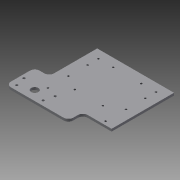
# Autodesk Inventor part: backplate
Saved by Autodesk Inventor 2013 (Build 170138000, 138)
## iProperties
Created: 2012-12-03
Part Number: backplate
Material: Generic
Document SubType Name: Sheet Metal
Designer: Istvan
Density: 1 g/cm^3
Sheet Metal Rule: Default
Flat Pattern Width: 24.13 cm
Flat Pattern Length: 20.32 cm
Flat Pattern Area: 490.322 cm^2
Sheet Metal Width: 9.500 in
Sheet Metal Length: 8.000 in
Sheet Metal Area: 76.000 in^2
Mass: 348.987 g
Surface Area: 1192.6 cm^2
Volume: 348.987 cm^3
Author: Istvan
Autodesk Inventor part; units mm, degrees
ref_plane "YZ Plane" through (0, 0, 0) normal (1, 0, 0) x (0, 1, 0)
ref_plane "XZ Plane" through (0, 0, 0) normal (0, 1, 0) x (-1, 0, 0)
ref_plane "XY Plane" through (0, 0, 0) normal (0, 0, 1) x (1, 0, 0)
sketch "Sketch1" plane through (0, 0, 0) normal (0, 1, 0) x (-1, 0, 0)
  line L0 (0, 0) -> (203.2, 0)
  line L1 (203.2, 0) -> (203.2, 114.3)
  line L2 (76.2, 165.1) -> (0, 165.1)
  line L3 (0, 165.1) -> (0, 0)
  line L4 (76.2, 165.1) -> (76.2, 190.5)
  line L5 (88.9, 203.2) -> (228.6, 203.2)
  arc A0 (63.5, 165.1) -> (76.2, 177.8) centre (63.5, 177.8) ccw
  arc A1 (241.3, 190.5) -> (228.6, 203.2) centre (228.6, 190.5) ccw
  arc A2 (88.9, 203.2) -> (76.2, 190.5) centre (88.9, 190.5) ccw
  line L6 (146.05, 0) -> (57.15, 0)
  line L7 (215.9, 127) -> (228.6, 127)
  line L8 (241.3, 139.7) -> (241.3, 190.5)
  arc A3 (215.9, 127) -> (203.2, 114.3) centre (215.9, 114.3) ccw
  arc A4 (228.6, 127) -> (241.3, 139.7) centre (228.6, 139.7) ccw
  point P0 (76.2, 203.2)
  point P1 (241.3, 127)
  dimension "d64" = 38.1
  dimension "d67" = 12.7
  dimension "d69" = 12.7
  dimension "d105" = 76.2
  dimension "d106" = 12.7
  dimension "d108" = 203.2
  dimension "d109" = 127
  dimension "d110" = 165.1
  dimension "d111" = 38.1
  constraints: 18 end point, 10 point on circle, 10 tangent, 6 point on line, 5 centre point, 3 horizontal, 2 equal radius, 2 parallel, 2 perpendicular, 1 midpoint
  measures "d64" distance of L2.start point (76.2, 203.2)
  measures "d67" radius of A0
  measures "d69" radius of A1
  measures "d105" distance between parallel lines of L3 L4
  measures "d106" radius of A3
  measures "d108" distance between parallel lines of L1 L3
  measures "d109" distance between parallel lines of L0 L7
  measures "d110" distance from line of L0.start L2
  measures "d111" distance between parallel lines of L8 L1
extrude "Plate2" add sketch "Sketch1" along normal blind 6.35
sketch "Sketch5" plane through (0, 6.35, 0) normal (0, 1, 0) x (1, 0, 0)
  line L0 (-203.2, -114.3) -> (-203.2, 0) projected
  line L1 (0, 0) -> (0, -165.1) projected
  line L2 (-203.2, 0) -> (0, 0) projected
  point P0 (-203.2, -165.1)
  point P1 (-177.8, -22.225)
  point P2 (-25.4, -22.225)
  point P3 (-25.4, -155.575)
  point P4 (-177.8, -155.575)
  point P5 (-177.8, -50.8)
  point P6 (-177.8, -101.6)
  point P7 (-25.4, -50.8)
  point P8 (-25.4, -101.6)
  point P9 (-203.2, -203.2)
  point P10 (-138.684, -22.225)
  point P11 (-64.516, -22.225)
  point P12 (-138.684, -123.825)
  point P13 (-64.516, -123.825)
  dimension "d27" = 25.4
  dimension "d28" = 25.4
  dimension "d30" = 133.35
  dimension "d62" = 22.225
  dimension "d89" = 50.8
  dimension "d90" = 50.8
  dimension "d91" = 25.4
  dimension "d93" = 152.4
  dimension "d94" = 25.4
  dimension "d147" = 64.516
  dimension "d148" = 64.516
  dimension "d149" = 101.6
  constraints: 7 horizontal alignment, 6 vertical alignment
  measures "d27" distance from line of L0 point (-177.8, -22.225)
  measures "d28" distance from line of L1 point (-25.4, -22.225)
  measures "d30" distance of point (-177.8, -155.575) point (-177.8, -22.225)
  measures "d62" distance from line of L2 point (-177.8, -22.225)
  measures "d89" distance from line of L2 point (-177.8, -50.8)
  measures "d90" distance of point (-177.8, -50.8) point (-177.8, -101.6)
  measures "d91" distance from line of L0 point (-177.8, -101.6)
  measures "d93" distance of point (-25.4, -50.8) point (-177.8, -50.8)
  measures "d94" distance from line of L1 point (-25.4, -50.8)
  measures "d147" distance from line of point (-138.684, -22.225) L0
  measures "d148" distance from line of point (-64.516, -22.225) L1
  measures "d149" distance of point (-138.684, -123.825) point (-138.684, -22.225)
hole "Hole2" at (-177.8, 6.35, 22.225) at (-25.4, 6.35, 22.225) at (-25.4, 6.35, 155.575) at (-177.8, 6.35, 155.575) at (-177.8, 6.35, 101.6) at (-177.8, 6.35, 50.8) at (-25.4, 6.35, 50.8) at (-25.4, 6.35, 101.6) at (-64.516, 6.35, 123.825) at (-138.684, 6.35, 123.825) at (-138.684, 6.35, 22.225) at (-64.516, 6.35, 22.225) direction (0, -1, 0) diameter 4.9784 end through all thread size "1/4-20 UNC" class "2B" standard "ANSI Unified Screw Threads"
sketch "Sketch12" plane through (0, 6.35, 0) normal (0, 1, 0) x (1, 0, 0)
  line L0 (-241.3, -190.5) -> (-241.3, -139.7) projected
  line L1 (-228.6, -127) -> (-215.9, -127) projected
  point P0 (-203.2, -203.2)
  point P1 (-190.5, -177.8)
  dimension "d107" = 50.8
  dimension "d129" = 50.8
  measures "d107" distance from line of L0 point (-190.5, -177.8)
  measures "d129" distance from line of point (-190.5, -177.8) L1
hole "Hole3" at (-190.5, 6.35, 177.8) direction (0, -1, 0) diameter 19.05 end through all
sketch "Sketch14" plane through (0, 6.35, 0) normal (0, 1, 0) x (1, 0, 0)
  circle A0 centre (-190.5, -177.8) radius 9.525 projected
  point P0 (0, 0)
  point P1 (-225.425, -190.5)
  point P2 (-155.575, -190.5)
  point P3 (-149.225, -165.1)
  point P4 (-231.775, -165.1)
  dimension "d130" = 6.35
  dimension "d135" = 6.35
  dimension "d136" = 25.4
  dimension "d137" = 12.7
  dimension "d138" = 82.55
  dimension "d139" = 41.275
  constraints: 2 horizontal alignment
  measures "d130" horizontal distance of point (-149.225, -165.1) point (-155.575, -190.5)
  measures "d135" horizontal distance of point (-231.775, -165.1) point (-225.425, -190.5)
  measures "d136" vertical distance of point (-149.225, -165.1) point (-155.575, -190.5)
  measures "d137" vertical distance of point (-149.225, -165.1) A0.centre
  measures "d138" distance of point (-149.225, -165.1) point (-231.775, -165.1)
  measures "d139" horizontal distance of A0.centre point (-149.225, -165.1)
hole "Hole5" at (-225.425, 6.35, 190.5) at (-155.575, 6.35, 190.5) at (-149.225, 6.35, 165.1) at (-231.775, 6.35, 165.1) direction (0, -1, 0) diameter 6.35 end through all
equation "\"d91\" = d94"
equation "\"d148\" = d147"
equation "\"d102\" = Thickness"
equation "\"d135\" = d130"
equation "\"d139\" = 0.5 * d138"
equation "\"d145\" = Thickness"
equation "\"d106\" = d69"
equation "\"BendRadius\" = Thickness"
equation "\"BendReliefWidth\" = Thickness"
equation "\"BendReliefDepth\" = 0.5 * Thickness"
equation "\"CornerReliefSize\" = 4 * Thickness"
equation "\"MinimumRemnant\" = 2 * Thickness"
equation "\"TransitionRadius\" = BendRadius"
equation "\"JacobiRadiusSize\" = Thickness"
equation "\"GapSize\" = Thickness"
equation "\"d15\" = BendRadius"
equation "\"d16\" = BendRadius"
equation "\"Thickness\" = 6.35"
body "Solid2"
